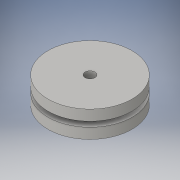
# Autodesk Inventor part: Wheel_design
Saved by Autodesk Inventor 2016 (Build 200138000, 138)
## iProperties
Created: 2016-02-28
Part Number: Wheel_design
Material: Generic
Document SubType Name: Modeling
Designer: torti_000
Density: 1 g/cm^3
Appearance: Default
Author: torti_000
Autodesk Inventor part; units mm, degrees
ref_plane "YZ Plane" through (0, 0, 0) normal (1, 0, 0) x (0, 1, 0)
ref_plane "XZ Plane" through (0, 0, 0) normal (0, 1, 0) x (-1, 0, 0)
ref_plane "XY Plane" through (0, 0, 0) normal (0, 0, 1) x (1, 0, 0)
sketch "Sketch1" plane through (0, 0, 0) normal (0, 1, 0) x (-1, 0, 0)
  circle A0 centre (0, 0) radius 25.4
  dimension "d0" = 50.8
  constraints: 1 centre point, 1 coincident
  measures "d0" diameter of A0
extrude "Extrusion1" add sketch "Sketch1" along normal blind 6.35
sketch "Sketch2" plane through (0, 6.35, 0) normal (0, 1, 0) x (1, 0, 0)
  circle A0 centre (0, 0) radius 19.05
  dimension "d3" = 38.1
  constraints: 1 centre point, 1 coincident
  measures "d3" diameter of A0
extrude "Extrusion2" add sketch "Sketch2" along normal blind 3.175
sketch "Sketch3" plane through (0, 9.525, 0) normal (0, 1, 0) x (1, 0, 0)
  circle A0 centre (0, 0) radius 25.4
  constraints: 1 centre point, 1 coincident
extrude "Extrusion3" add sketch "Sketch3" along normal blind 6.35
sketch "Sketch5" plane through (0, 15.875, 0) normal (0, 1, 0) x (1, 0, 0)
  circle A0 centre (0, 0) radius 3
  dimension "d10" = 6
  constraints: 1 centre point, 1 coincident
  measures "d10" diameter of A0
hole "Hole1" at (0, 15.875, 0) direction (0, -1, 0) diameter 6 end through all
body "Solid1"
